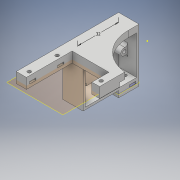
# Autodesk Inventor part: imu_holder
Saved by Autodesk Inventor 2018 (Build 220112000, 112)
## iProperties
Created: 2020-02-18
Part Number: imu_holder
Material: Generic
Document SubType Name: Modeling
Designer: bitbots
Density: 1 g/cm^3
Appearance: Default
Author: bitbots
Autodesk Inventor part; units mm, degrees
ref_plane "YZ Plane" through (0, 0, 0) normal (1, 0, 0) x (0, 1, 0)
ref_plane "XZ Plane" through (0, 0, 0) normal (0, 1, 0) x (-1, 0, 0)
ref_plane "XY Plane" through (0, 0, 0) normal (0, 0, 1) x (1, 0, 0)
sketch "Sketch1" plane through (0, 0, 0) normal (0, 0, 1) x (1, 0, 0)
  arc A0 (-19.5808, 6.2636) -> (-20.1, 4.5766) centre (-17.1, 4.5766) ccw projected
  line L0 (-20.1, -39.6766) -> (-20.1, 4.5766) projected
  arc A1 (-20.1, -39.6766) -> (-19.5808, -41.3636) centre (-17.1, -39.6766) ccw projected
  line L1 (-15.8929, -46.7869) -> (-19.5808, -41.3636) projected
  arc A2 (-15.8929, -46.7869) -> (-13.4121, -48.1) centre (-13.4121, -45.1) ccw projected
  line L2 (13.4121, -48.1) -> (-13.4121, -48.1) projected
  arc A3 (13.4121, -48.1) -> (15.8929, -46.7869) centre (13.4121, -45.1) ccw projected
  line L3 (19.5808, -41.3636) -> (15.8929, -46.7869) projected
  arc A4 (19.5808, -41.3636) -> (20.1, -39.6766) centre (17.1, -39.6766) ccw projected
  line L4 (20.1, 4.5766) -> (20.1, -39.6766) projected
  arc A5 (20.1, 4.5766) -> (19.5808, 6.2636) centre (17.1, 4.5766) ccw projected
  line L5 (15.5953, 12.1246) -> (19.5808, 6.2636) projected
  arc A6 (15.5953, 12.1246) -> (13.9414, 13) centre (13.9414, 11) ccw projected
  line L6 (7.65, 13) -> (13.9414, 13) projected
  arc A7 (9.15, 11.5) -> (7.65, 13) centre (7.65, 11.5) ccw projected
  line L7 (9.15, 11.5) -> (9.15, 10) projected
  arc A8 (9.15, 10) -> (11.5, 7.65) centre (11.5, 10) ccw projected
  line L8 (11.5, 7.65) -> (13.5, 7.65) projected
  arc A9 (14.5, 6.65) -> (13.5, 7.65) centre (13.5, 6.65) ccw projected
  line L9 (14.5, 6.65) -> (14.5, -36.15) projected
  arc A10 (13.5, -37.15) -> (14.5, -36.15) centre (13.5, -36.15) ccw projected
  line L10 (13.5, -37.15) -> (11.5, -37.15) projected
  arc A11 (11.5, -37.15) -> (9.15, -39.5) centre (11.5, -39.5) ccw projected
  line L11 (9.15, -39.5) -> (9.15, -41.5) projected
  arc A12 (8.15, -42.5) -> (9.15, -41.5) centre (8.15, -41.5) ccw projected
  line L12 (8.15, -42.5) -> (-8.15, -42.5) projected
  arc A13 (-9.15, -41.5) -> (-8.15, -42.5) centre (-8.15, -41.5) ccw projected
  line L13 (-9.15, -41.5) -> (-9.15, -39.5) projected
  arc A14 (-9.15, -39.5) -> (-11.5, -37.15) centre (-11.5, -39.5) ccw projected
  line L14 (-11.5, -37.15) -> (-13.5, -37.15) projected
  arc A15 (-14.5, -36.15) -> (-13.5, -37.15) centre (-13.5, -36.15) ccw projected
  line L15 (-14.5, -36.15) -> (-14.5, 6.65) projected
  arc A16 (-13.5, 7.65) -> (-14.5, 6.65) centre (-13.5, 6.65) ccw projected
  line L16 (-13.5, 7.65) -> (-11.5, 7.65) projected
  arc A17 (-11.5, 7.65) -> (-9.15, 10) centre (-11.5, 10) ccw projected
  line L17 (-9.15, 10) -> (-9.15, 11.5) projected
  arc A18 (-7.65, 13) -> (-9.15, 11.5) centre (-7.65, 11.5) ccw projected
  line L18 (-13.9414, 13) -> (-7.65, 13) projected
  arc A19 (-13.9414, 13) -> (-15.5953, 12.1246) centre (-13.9414, 11) ccw projected
  line L19 (-19.5808, 6.2636) -> (-15.5953, 12.1246) projected
  circle A20 centre (17.3, 4) radius 1.35 projected
  circle A21 centre (17.3, -18) radius 1.35 projected
  circle A22 centre (11, -45.3) radius 1.35 projected
  circle A23 centre (-17.3, 4) radius 1.35 projected
  circle A24 centre (-17.3, -18) radius 1.35 projected
  circle A25 centre (-11, -45.3) radius 1.35 projected
  circle A26 centre (17.3, -40) radius 1.35 projected
  circle A27 centre (-17.3, -40) radius 1.35 projected
  line L20 (-17.3, -18) -> (-17.3, -23)
  line L21 (-17.3, -18) -> (-12.3, -18) construction
  line L22 (-17.3, -23) -> (-14.5, -23)
  line L23 (-14.5, -23) -> (-22.5, -23)
  line L24 (-22.5, -23) -> (-22.5, 13.5)
  line L25 (-22.5, 13.5) -> (-14.5, 13.5)
  line L26 (-14.5, 13.5) -> (-14.5, -23)
  line L27 (0, 0) -> (0, -50) construction
  line L28 (14.5, -23) -> (22.5, -23)
  line L29 (22.5, -23) -> (22.5, 13.5)
  line L30 (22.5, 13.5) -> (14.5, 13.5)
  line L31 (14.5, 13.5) -> (14.5, -23)
  line L32 (7.65, 13) -> (-7.65, 13) construction
  line L33 (14.5, 13.5) -> (-14.5, 13.5)
  line L34 (-14.5, 13.5) -> (-14.5, 12.9204)
  line L35 (-14.5, 12.9204) -> (14.5, 12.9204)
  line L36 (14.5, 12.9204) -> (14.5, 13.5)
  dimension "d0" = 5
  dimension "d1" = 90
  dimension "d2" = 8
  dimension "d3" = 36.5
  dimension "d4" = 50
  constraints: 32 end point, 4 parallel, 4 perpendicular, 4 symmetric about line, 3 horizontal, 2 point on line, 2 vertical, 1 point on circle
  measures "d0" distance of L20.start L20.end
  measures "d1" angle of L20 L21
  measures "d2" distance of L24.end L25.end
  measures "d3" distance of L23.end L24.end
  measures "d4" distance of L27.start L27.end
ref_plane "Work Plane1" through (-4.0114, -4.0114, 5) normal (0, 0, 1) x (1, 0, 0)
extrude "Extrusion1" add sketch "Sketch1" along normal up to surface (5 mm away) contours L19 A19 L26 L15 L22 L23 L0 A0 | A0 L0 L23 L24 L25 L26 A19 L19 | L26 L33 L31 A6 L6 A7 L35 A18 L18 A19 | A19 L18 A18 L35 | L30 L29 L28 L4 A5 L5 A6 L31 | A7 L6 A6 L35 | A6 L5 A5 L4 L28 L9 L31
ref_plane "Work Plane2" through (-22.5, 13.5, 2.5) normal (0, 0, 1) x (1, 0, 0)
sketch "Sketch3" plane through (-22.5, 13.5, 2.5) normal (0, 0, 1) x (1, 0, 0)
  line L0 (37, -36.5) -> (37, -0.5796) projected
  line L1 (45, -36.5) -> (37, -36.5) projected
  line L2 (45, 0) -> (45, -36.5) projected
  line L3 (0, 0) -> (45, 0) projected
  line L4 (0, -36.5) -> (0, 0) projected
  line L5 (8, -36.5) -> (0, -36.5) projected
  line L6 (8, -0.5796) -> (8, -36.5) projected
  line L7 (37, -0.5796) -> (8, -0.5796) projected
  circle A0 centre (39.8, -9.5) radius 1.35 projected
  circle A1 centre (39.8, -31.5) radius 1.35 projected
  circle A2 centre (5.2, -9.5) radius 1.35 projected
  circle A3 centre (5.2, -31.5) radius 1.35 projected
  line L8 (2.4, -29.025) -> (8, -29.025)
  line L9 (8, -29.025) -> (8, -33.975)
  line L10 (8, -33.975) -> (2.4, -33.975)
  line L11 (2.4, -33.975) -> (2.4, -29.025)
  line L12 (2.4, -29.025) -> (8, -33.975) construction
  line L13 (8, -29.025) -> (2.4, -33.975) construction
  line L14 (2.4, -7.025) -> (8, -7.025)
  line L15 (8, -7.025) -> (8, -11.975)
  line L16 (8, -11.975) -> (2.4, -11.975)
  line L17 (2.4, -11.975) -> (2.4, -7.025)
  line L18 (2.4, -7.025) -> (8, -11.975) construction
  line L19 (8, -7.025) -> (2.4, -11.975) construction
  line L20 (37, -7.025) -> (42.6, -7.025)
  line L21 (42.6, -7.025) -> (42.6, -11.975)
  line L22 (42.6, -11.975) -> (37, -11.975)
  line L23 (37, -11.975) -> (37, -7.025)
  line L24 (37, -7.025) -> (42.6, -11.975) construction
  line L25 (42.6, -7.025) -> (37, -11.975) construction
  line L26 (37, -29.025) -> (42.6, -29.025)
  line L27 (42.6, -29.025) -> (42.6, -33.975)
  line L28 (42.6, -33.975) -> (37, -33.975)
  line L29 (37, -33.975) -> (37, -29.025)
  line L30 (37, -29.025) -> (42.6, -33.975) construction
  line L31 (42.6, -29.025) -> (37, -33.975) construction
  point P0 (22.5, -13.5)
  dimension "d16" = 5.6
  dimension "d17" = 4.95
  dimension "d18" = 5.6
  dimension "d19" = 4.95
  dimension "d20" = 5.6
  dimension "d21" = 4.95
  dimension "d22" = 5.6
  dimension "d23" = 4.95
  constraints: 48 end point, 8 midpoint, 8 parallel, 4 horizontal, 4 perpendicular
  measures "d16" distance of L9.end L10.end
  measures "d17" distance of L8.end L9.end
  measures "d18" distance of L15.end L16.end
  measures "d19" distance of L14.end L15.end
  measures "d20" distance of L21.end L22.end
  measures "d21" distance of L20.end L21.end
  measures "d22" distance of L27.end L28.end
  measures "d23" distance of L26.end L27.end
extrude "Extrusion2" cut sketch "Sketch3" along normal blind 1.6 contours L0 L26 L27 L28 | L0 L20 L21 L22 | L10 L11 L8 L6 | L6 L16 L17 L14
sketch "Sketch4" plane through (-22.5, 13.5, 0) normal (0, 1, 0) x (1, 0, 0)
  line L0 (0, -5) -> (45, -5) construction
  line L1 (45, 0) -> (45, -5) construction
  line L2 (45, 0) -> (0, 0) construction
  line L3 (0, 0) -> (0, -5) construction
  line L4 (0, 0) -> (0, -5) projected
  line L5 (0, -5) -> (16, -5)
  line L6 (16, -5) -> (16, 29)
  line L7 (16, 29) -> (0, 29)
  line L8 (0, 29) -> (0, -5)
  point P0 (22.5, 0)
  dimension "d26" = 16
  dimension "d27" = 34
  constraints: 8 end point, 2 parallel, 1 horizontal, 1 perpendicular
  measures "d26" distance of L7.end L6.end
  measures "d27" distance of L6.end L5.end
extrude "Extrusion3" add sketch "Sketch4" along normal blind 44
sketch "Sketch5" plane through (-22.5, -23, 0) normal (-1, 0, 0) x (0, 0, 1)
  line L0 (5, 0) -> (5, 80.5) construction
  line L1 (-29, 80.5) -> (5, 80.5) construction
  line L2 (-29, 36.5) -> (-29, 80.5) construction
  line L3 (-29, 36.5) -> (0, 36.5) construction
  line L4 (0, 36.5) -> (0, 0) construction
  line L5 (0, 0) -> (5, 0) construction
  line L6 (-29, 80.5) -> (5, 80.5) construction
  line L7 (5, 80.5) -> (5, 65.6) construction
  line L8 (5, 0) -> (5, 80.5) construction
  line L9 (5, 80.5) -> (19.9, 80.5) construction
  line L10 (5, 65.6) -> (-2.5, 65.6) construction
  line L11 (-2.5, 65.6) -> (-12, 65.6) construction
  line L12 (-12, 65.6) -> (-21.5, 65.6) construction
  line L13 (-0.2, 63.3) -> (-4.8, 63.3)
  line L14 (-4.8, 63.3) -> (-4.8, 67.9)
  line L15 (-4.8, 67.9) -> (-0.2, 67.9)
  line L16 (-0.2, 67.9) -> (-0.2, 63.3)
  line L17 (-0.2, 63.3) -> (-4.8, 67.9) construction
  line L18 (-4.8, 63.3) -> (-0.2, 67.9) construction
  line L19 (-9.7, 63.3) -> (-14.3, 63.3)
  line L20 (-14.3, 63.3) -> (-14.3, 67.9)
  line L21 (-14.3, 67.9) -> (-9.7, 67.9)
  line L22 (-9.7, 67.9) -> (-9.7, 63.3)
  line L23 (-9.7, 63.3) -> (-14.3, 67.9) construction
  line L24 (-14.3, 63.3) -> (-9.7, 67.9) construction
  line L25 (-19.2, 63.3) -> (-23.8, 63.3)
  line L26 (-23.8, 63.3) -> (-23.8, 67.9)
  line L27 (-23.8, 67.9) -> (-19.2, 67.9)
  line L28 (-19.2, 67.9) -> (-19.2, 63.3)
  line L29 (-19.2, 63.3) -> (-23.8, 67.9) construction
  line L30 (-23.8, 63.3) -> (-19.2, 67.9) construction
  point P0 (0, 23)
  dimension "d30" = 14.9
  dimension "d31" = 90
  dimension "d32" = 7.5
  dimension "d33" = 90
  dimension "d34" = 9.5
  dimension "d35" = 9.5
  dimension "d36" = 4.6
  dimension "d37" = 4.6
  dimension "d38" = 4.6
  dimension "d39" = 4.6
  dimension "d40" = 4.6
  dimension "d41" = 4.6
  constraints: 46 end point, 6 midpoint, 6 parallel, 5 perpendicular, 4 horizontal, 2 point on line, 1 collinear
  measures "d30" distance of L0.end L7.end
  measures "d31" angle of L7 L9
  measures "d32" distance of L7.end L10.end
  measures "d33" angle of L7 L10
  measures "d34" distance of L10.end L11.end
  measures "d35" distance of L11.end L12.end
  measures "d36" distance of L14.end L15.end
  measures "d37" distance of L13.end L14.end
  measures "d38" distance of L20.end L21.end
  measures "d39" distance of L19.end L20.end
  measures "d40" distance of L26.end L27.end
  measures "d41" distance of L25.end L26.end
extrude "Extrusion4" cut sketch "Sketch5" against normal blind 9
sketch "Sketch6" plane through (-22.5, 57.5, 0) normal (0, 1, 0) x (1, 0, 0)
  line L0 (0, -5) -> (16, -5) construction
  line L1 (16, -5) -> (16, 29) construction
  line L2 (16, 29) -> (0, 29) construction
  line L3 (0, 29) -> (0, -5) construction
  point P0 (22.5, 0)
sketch "Sketch7" plane through (-6.5, 13.5, 0) normal (1, 0, 0) x (0, 0, -1)
  line L0 (-5, 44) -> (29, 44) projected
  line L1 (-5, 44) -> (-5, 42.2)
  line L2 (-5, 0) -> (-5, 44) projected
  line L3 (-5, 42.2) -> (-3.2, 42.2)
  line L4 (-3.2, 42.2) -> (27.2, 42.2)
  line L5 (27.2, 42.2) -> (27.2, 1.8)
  line L6 (27.2, 1.8) -> (-3.2, 1.8)
  line L7 (-3.2, 1.8) -> (-3.2, 42.2)
  point P0 (0, -13.5)
  dimension "d44" = 1.8
  dimension "d45" = 1.8
  dimension "d46" = 90
  dimension "d47" = 30.4
  dimension "d48" = 40.4
  constraints: 12 end point, 2 parallel, 2 perpendicular, 1 horizontal, 1 point on line
  measures "d44" distance of L0.start L1.end
  measures "d45" distance of L1.end L3.end
  measures "d46" angle of L3 L1
  measures "d47" distance of L5.end L6.end
  measures "d48" distance of L4.end L5.end
extrude "Extrusion5" cut sketch "Sketch7" against normal blind 14
sketch "Sketch8" plane through (-20.5, 13.5, 0) normal (1, 0, 0) x (0, 0, -1)
  line L0 (9.7, 31.4) -> (9.7, 26.8) construction
  line L1 (14.3, 31.4) -> (9.7, 31.4) construction
  line L2 (14.3, 26.8) -> (14.3, 31.4) construction
  line L3 (9.7, 26.8) -> (14.3, 26.8) construction
  line L4 (0.2, 31.4) -> (0.2, 26.8) construction
  line L5 (4.8, 31.4) -> (0.2, 31.4) construction
  line L6 (4.8, 26.8) -> (4.8, 31.4) construction
  line L7 (0.2, 26.8) -> (4.8, 26.8) construction
  line L8 (19.2, 31.4) -> (19.2, 26.8) construction
  line L9 (23.8, 31.4) -> (19.2, 31.4) construction
  line L10 (23.8, 26.8) -> (23.8, 31.4) construction
  line L11 (19.2, 26.8) -> (23.8, 26.8) construction
  line L12 (-3.2, 1.8) -> (-3.2, 42.2) construction
  line L13 (27.2, 1.8) -> (-3.2, 1.8) construction
  line L14 (27.2, 42.2) -> (27.2, 1.8) construction
  line L15 (-3.2, 42.2) -> (27.2, 42.2) construction
  line L16 (27.2, 1.8) -> (-3.2, 1.8) construction
  line L17 (-3.2, 1.8) -> (1.65, 1.8) construction
  line L18 (-3.2, 1.8) -> (1.65, 1.8) construction
  line L19 (1.65, 1.8) -> (1.65, 4.6) construction
  line L20 (1.65, 4.6) -> (21.95, 4.6) construction
  circle A0 centre (1.65, 4.6) radius 1.35
  circle A1 centre (21.95, 4.6) radius 1.35
  circle A2 centre (21.95, 4.6) radius 2.9
  circle A3 centre (1.65, 4.6) radius 2.9
  line L21 (-3.2, 42.2) -> (27.2, 42.2) projected
  line L22 (-3.2, 42.2) -> (11.8, 42.2)
  line L23 (-3.2, 42.2) -> (11.8, 42.2) construction
  line L24 (11.8, 42.2) -> (11.8, 39.5)
  circle A4 centre (11.8, 39.5) radius 1.35
  circle A5 centre (11.8, 39.5) radius 2.6
  point P0 (0, -13.5)
  dimension "d51" = 4.85
  dimension "d52" = 0
  dimension "d53" = 2.8
  dimension "d54" = 90
  dimension "d55" = 20.3
  dimension "d56" = 90
  dimension "d57" = 2.7
  dimension "d58" = 2.7
  dimension "d59" = 5.8
  dimension "d60" = 5.8
  dimension "d61" = 15
  dimension "d62" = 0
  dimension "d63" = 2.7
  dimension "d64" = 2.7
  dimension "d65" = 5.2
  constraints: 14 end point, 6 centre point, 6 coincident, 4 collinear, 3 perpendicular, 2 horizontal
  measures "d51" distance of L12.start L17.end
  measures "d52" distance between parallel lines of L18 L17
  measures "d53" distance of L17.end L19.end
  measures "d54" angle of L19 L17
  measures "d55" distance of L19.end L20.end
  measures "d56" angle of L19 L20
  measures "d57" diameter of A0
  measures "d58" diameter of A1
  measures "d59" diameter of A2
  measures "d60" diameter of A3
  measures "d61" distance of L12.end L22.end
  measures "d62" distance between parallel lines of L23 L22
  measures "d63" distance of L22.end L24.end
  measures "d64" diameter of A4
  measures "d65" diameter of A5
extrude "Extrusion6" cut sketch "Sketch8" against normal up to surface (2 mm away) contours A0 | A1 | A4
sketch "Sketch10" plane through (-20.5, 13.5, 0) normal (1, 0, 0) x (0, 0, -1)
  circle A0 centre (1.65, 4.6) radius 1.35 construction
  circle A1 centre (11.8, 39.5) radius 1.35 projected
  circle A2 centre (21.95, 4.6) radius 1.35 projected
  line L0 (9.7, 31.4) -> (9.7, 26.8) construction
  line L1 (14.3, 31.4) -> (9.7, 31.4) construction
  line L2 (14.3, 26.8) -> (14.3, 31.4) construction
  line L3 (9.7, 26.8) -> (14.3, 26.8) construction
  line L4 (0.2, 31.4) -> (0.2, 26.8) construction
  line L5 (4.8, 31.4) -> (0.2, 31.4) construction
  line L6 (4.8, 26.8) -> (4.8, 31.4) construction
  line L7 (0.2, 26.8) -> (4.8, 26.8) construction
  line L8 (19.2, 31.4) -> (19.2, 26.8) construction
  line L9 (23.8, 31.4) -> (19.2, 31.4) construction
  line L10 (23.8, 26.8) -> (23.8, 31.4) construction
  line L11 (19.2, 26.8) -> (23.8, 26.8) construction
  line L12 (-3.2, 1.8) -> (-3.2, 42.2) construction
  line L13 (27.2, 1.8) -> (-3.2, 1.8) construction
  line L14 (27.2, 42.2) -> (27.2, 1.8) construction
  line L15 (-3.2, 42.2) -> (27.2, 42.2) construction
  circle A3 centre (11.8, 39.5) radius 2.75
  circle A4 centre (21.95, 4.6) radius 2.85
  circle A5 centre (1.65, 4.6) radius 1.35 projected
  circle A6 centre (1.65, 4.6) radius 2.85
  point P0 (0, -13.5)
  dimension "d68" = 5.5
  dimension "d69" = 5.7
  dimension "d70" = 5.7
  constraints: 3 centre point, 3 coincident
  measures "d68" diameter of A3
  measures "d69" diameter of A4
  measures "d70" diameter of A6
extrude "Extrusion7" add sketch "Sketch10" along normal blind 7
sketch "Sketch11" plane through (-22.5, -23, 0) normal (-1, 0, 0) x (0, 0, 1)
  line L0 (5, 0) -> (5, 80.5) construction
  line L1 (-29, 80.5) -> (5, 80.5) construction
  line L2 (-29, 36.5) -> (-29, 80.5) construction
  line L3 (-29, 36.5) -> (0, 36.5) construction
  line L4 (0, 36.5) -> (0, 0) construction
  line L5 (0, 0) -> (5, 0) construction
  line L6 (0.85, 38.6) -> (-4.15, 38.6)
  line L7 (-4.15, 38.6) -> (-4.15, 43.6)
  line L8 (-4.15, 43.6) -> (0.85, 43.6)
  line L9 (0.85, 43.6) -> (0.85, 38.6)
  line L10 (0.85, 38.6) -> (-4.15, 43.6) construction
  line L11 (-4.15, 38.6) -> (0.85, 43.6) construction
  line L12 (-19.45, 38.6) -> (-24.45, 38.6)
  line L13 (-24.45, 38.6) -> (-24.45, 43.6)
  line L14 (-24.45, 43.6) -> (-19.45, 43.6)
  line L15 (-19.45, 43.6) -> (-19.45, 38.6)
  circle A0 centre (-21.95, 41.1) radius 1.35 projected
  line L16 (-19.45, 38.6) -> (-24.45, 43.6) construction
  line L17 (-24.45, 38.6) -> (-19.45, 43.6) construction
  line L18 (-9.3, 73.5) -> (-14.3, 73.5)
  line L19 (-14.3, 73.5) -> (-14.3, 78.5)
  line L20 (-14.3, 78.5) -> (-9.3, 78.5)
  line L21 (-9.3, 78.5) -> (-9.3, 73.5)
  circle A1 centre (-11.8, 76) radius 1.35 projected
  line L22 (-9.3, 73.5) -> (-14.3, 78.5) construction
  line L23 (-14.3, 73.5) -> (-9.3, 78.5) construction
  circle A2 centre (-1.65, 41.1) radius 1.35 construction
  point P0 (0, 23)
  dimension "d73" = 5
  dimension "d74" = 5
  dimension "d75" = 5
  dimension "d76" = 5
  dimension "d77" = 5
  dimension "d78" = 5
  constraints: 36 end point, 6 parallel, 5 midpoint, 3 horizontal, 3 perpendicular, 1 coincident
  measures "d73" distance of L7.end L8.end
  measures "d74" distance of L6.end L7.end
  measures "d75" distance of L13.end L14.end
  measures "d76" distance of L12.end L13.end
  measures "d77" distance of L19.end L20.end
  measures "d78" distance of L18.end L19.end
extrude "Extrusion8" cut sketch "Sketch11" against normal blind 1.6
sketch "Sketch12" plane through (-22.5, -23, 0) normal (-1, 0, 0) x (0, 0, 1)
  line L0 (-14.3, 78.5) -> (-9.3, 78.5) construction
  line L1 (5, 0) -> (5, 80.5) construction
  line L2 (-29, 80.5) -> (5, 80.5) construction
  line L3 (-29, 36.5) -> (-29, 80.5) construction
  line L4 (-29, 36.5) -> (0, 36.5) construction
  line L5 (0, 36.5) -> (0, 0) construction
  line L6 (0, 0) -> (5, 0) construction
  line L7 (5, 36.5) -> (5, 80.5) construction
  line L8 (5, 80.5) -> (5, 48.5) construction
  line L9 (-9.3, 78.5) -> (-9.3, 73.5) projected
  line L10 (-9.3, 73.5) -> (-14.3, 73.5) projected
  line L11 (-14.3, 73.5) -> (-14.3, 78.5) projected
  point P0 (0, 23)
  dimension "d81" = 32
  constraints: 2 end point, 1 point on line
  measures "d81" distance of L1.end L8.end
ref_plane "Work Plane3" through (-24.5, -41.5055, -34.0037) normal (1, 0, 0) x (0, 1, 0)
sketch "Sketch14" plane through (-6.5, 13.5, -29) normal (0, 0, -1) x (-1, 0, 0)
  line L0 (23, -53) -> (5.6855, -75.3568) construction
  line L1 (23, -53) -> (23, 42.8925) construction
  arc A0 (23, 42.8925) -> (22.4142, 44.3067) centre (21, 42.8925) ccw construction
  line L2 (22.4142, 44.3067) -> (9.3067, 57.4142) construction
  arc A1 (9.3067, 57.4142) -> (7.8925, 58) centre (7.8925, 56) ccw construction
  line L3 (7.8925, 58) -> (-5.1716, 58) construction
  arc A2 (-5.1716, 58) -> (-6.5858, 57.4142) centre (-5.1716, 56) ccw construction
  line L4 (-6.5858, 57.4142) -> (-11.4142, 52.5858) construction
  arc A3 (-12.8284, 52) -> (-11.4142, 52.5858) centre (-12.8284, 54) ccw construction
  line L5 (-12.8284, 52) -> (-127, 52) construction
  line L6 (-127, 52) -> (-127, -73) construction
  line L7 (-127, -73) -> (-121.462, -73) construction
  arc A4 (-120.54, -73.0426) -> (-121.462, -73) centre (-121.462, -83) ccw construction
  line L8 (-120.54, -73.0426) -> (-67.46, -77.9574) construction
  arc A5 (-67.46, -77.9574) -> (-66.538, -78) centre (-66.538, -68) ccw construction
  line L9 (-66.538, -78) -> (-1.0877, -78) construction
  arc A6 (-1.0877, -78) -> (5.6855, -75.3568) centre (-1.0877, -68) ccw construction
  circle A7 centre (-73, 42) radius 2.5 construction
  circle A8 centre (-73, -13) radius 2.5 construction
  circle A9 centre (6, 39) radius 2.5 construction
  circle A10 centre (-11, 47) radius 2.5 construction
  circle A11 centre (-35.5, 47) radius 2.5 construction
  circle A12 centre (-60, 47) radius 2.5 construction
  circle A13 centre (-111, -69) radius 2.5 construction
  circle A14 centre (-77.1448, -72.1347) radius 2.5 construction
  circle A15 centre (-60, -73) radius 2.5 construction
  circle A16 centre (-35.5, -73) radius 2.5 construction
  circle A17 centre (-11, -73) radius 2.5 construction
  circle A18 centre (10.8, -53.5) radius 1.025 construction
  circle A19 centre (10.8, -31.5) radius 1.025 construction
  circle A20 centre (10.8, -9.5) radius 1.025 construction
  circle A21 centre (-23.8, -9.5) radius 1.025 construction
  circle A22 centre (-23.8, -31.5) radius 1.025 construction
  circle A23 centre (-23.8, -53.5) radius 1.025 construction
  circle A24 centre (4.5, -58.8) radius 1.025 construction
  circle A25 centre (-17.5, -58.8) radius 1.025 construction
  circle A26 centre (-73, -68) radius 2.5 construction
  line L10 (-28, 43) -> (-65.5, 43) construction
  arc A27 (-26, 41) -> (-28, 43) centre (-28, 41) ccw construction
  line L11 (-26, 41) -> (-26, 22) construction
  arc A28 (-28, 20) -> (-26, 22) centre (-28, 22) ccw construction
  line L12 (-28, 20) -> (-65.5, 20) construction
  arc A29 (-67.5, 22) -> (-65.5, 20) centre (-65.5, 22) ccw construction
  line L13 (-67.5, 22) -> (-67.5, 41) construction
  arc A30 (-65.5, 43) -> (-67.5, 41) centre (-65.5, 41) ccw construction
  line L14 (-118, 46.5) -> (-80.5, 46.5) construction
  arc A31 (-78.5, 44.5) -> (-80.5, 46.5) centre (-80.5, 44.5) ccw construction
  line L15 (-78.5, 44.5) -> (-78.5, 22) construction
  arc A32 (-80.5, 20) -> (-78.5, 22) centre (-80.5, 22) ccw construction
  line L16 (-80.5, 20) -> (-118, 20) construction
  arc A33 (-120, 22) -> (-118, 20) centre (-118, 22) ccw construction
  line L17 (-120, 22) -> (-120, 44.5) construction
  arc A34 (-118, 46.5) -> (-120, 44.5) centre (-118, 44.5) ccw construction
  line L18 (-111.9569, 15) -> (-80.5, 15) construction
  arc A35 (-78.5, 13) -> (-80.5, 15) centre (-80.5, 13) ccw construction
  line L19 (-78.5, 13) -> (-78.5, -21.3542) construction
  arc A36 (-81.975, -22.7049) -> (-78.5, -21.3542) centre (-80.5, -21.3542) ccw construction
  line L20 (-81.975, -22.7049) -> (-113.4319, 11.6494) construction
  arc A37 (-111.9569, 15) -> (-113.4319, 11.6494) centre (-111.9569, 13) ccw construction
  line L21 (-86.5431, -30) -> (-118, -30) construction
  arc A38 (-120, -28) -> (-118, -30) centre (-118, -28) ccw construction
  line L22 (-120, -28) -> (-120, 6.3542) construction
  arc A39 (-116.525, 7.7049) -> (-120, 6.3542) centre (-118, 6.3542) ccw construction
  line L23 (-116.525, 7.7049) -> (-85.0681, -26.6494) construction
  arc A40 (-86.5431, -30) -> (-85.0681, -26.6494) centre (-86.5431, -28) ccw construction
  line L24 (-64.025, 7.7049) -> (-32.5681, -26.6494) construction
  arc A41 (-34.0431, -30) -> (-32.5681, -26.6494) centre (-34.0431, -28) ccw construction
  line L25 (-34.0431, -30) -> (-65.5, -30) construction
  arc A42 (-67.5, -28) -> (-65.5, -30) centre (-65.5, -28) ccw construction
  line L26 (-67.5, -28) -> (-67.5, 6.3542) construction
  arc A43 (-64.025, 7.7049) -> (-67.5, 6.3542) centre (-65.5, 6.3542) ccw construction
  line L27 (-29.475, -22.7049) -> (-60.9319, 11.6494) construction
  arc A44 (-59.4569, 15) -> (-60.9319, 11.6494) centre (-59.4569, 13) ccw construction
  line L28 (-59.4569, 15) -> (-28, 15) construction
  arc A45 (-26, 13) -> (-28, 15) centre (-28, 13) ccw construction
  line L29 (-26, 13) -> (-26, -21.3542) construction
  arc A46 (-29.475, -22.7049) -> (-26, -21.3542) centre (-28, -21.3542) ccw construction
  line L30 (-67.5, -67) -> (-67.5, -37) construction
  arc A47 (-65.5, -35) -> (-67.5, -37) centre (-65.5, -37) ccw construction
  line L31 (-65.5, -35) -> (-28, -35) construction
  arc A48 (-26, -37) -> (-28, -35) centre (-28, -37) ccw construction
  line L32 (-26, -37) -> (-26, -67) construction
  arc A49 (-28, -69) -> (-26, -67) centre (-28, -67) ccw construction
  line L33 (-65.5, -69) -> (-28, -69) construction
  arc A50 (-67.5, -67) -> (-65.5, -69) centre (-65.5, -67) ccw construction
  line L34 (5.0579, 54.1421) -> (18.4929, 40.7071) construction
  arc A51 (18.4929, 39.2929) -> (18.4929, 40.7071) centre (17.7858, 40) ccw construction
  line L35 (18.4929, 39.2929) -> (17.7363, 38.5363) construction
  arc A52 (16.3221, 38.5363) -> (17.7363, 38.5363) centre (17.0292, 39.2434) ccw construction
  line L36 (16.3221, 38.5363) -> (2.887, 51.9713) construction
  arc A53 (2.887, 53.3855) -> (2.887, 51.9713) centre (3.5942, 52.6784) ccw construction
  line L37 (2.887, 53.3855) -> (3.6437, 54.1421) construction
  arc A54 (5.0579, 54.1421) -> (3.6437, 54.1421) centre (4.3508, 53.435) ccw construction
  line L38 (-120, -63) -> (-120, -37) construction
  arc A55 (-118, -35) -> (-120, -37) centre (-118, -37) ccw construction
  line L39 (-118, -35) -> (-80.5, -35) construction
  arc A56 (-78.5, -37) -> (-80.5, -35) centre (-80.5, -37) ccw construction
  line L40 (-78.5, -37) -> (-78.5, -68.3661) construction
  arc A57 (-78.636, -68.4231) -> (-78.5, -68.3661) centre (-80.5, -63.7835) ccw construction
  arc A58 (-78.636, -68.4231) -> (-80.5765, -70.0796) centre (-77.1448, -72.1347) ccw construction
  arc A59 (-82.4767, -71.0434) -> (-80.5765, -70.0796) centre (-82.2923, -69.052) ccw construction
  line L41 (-82.4767, -71.0434) -> (-105.5584, -68.9063) construction
  arc A60 (-107.2493, -67.6098) -> (-105.5584, -68.9063) centre (-105.374, -66.9148) ccw construction
  arc A61 (-107.2493, -67.6098) -> (-111, -65) centre (-111, -69) ccw construction
  line L42 (-111, -65) -> (-118, -65) construction
  arc A62 (-120, -63) -> (-118, -65) centre (-118, -63) ccw construction
  line L43 (0, 43) -> (-19, 43) construction
  arc A63 (2, 41) -> (0, 43) centre (0, 41) ccw construction
  line L44 (2, 41) -> (2, 39) construction
  arc A64 (2, 39) -> (6, 35) centre (6, 39) ccw construction
  line L45 (6, 35) -> (11, 35) construction
  arc A65 (16, 30) -> (11, 35) centre (11, 30) ccw construction
  line L46 (16, 30) -> (16, -3.5) construction
  arc A66 (14, -5.5) -> (16, -3.5) centre (14, -3.5) ccw construction
  line L47 (14, -5.5) -> (10, -5.5) construction
  arc A67 (10, -5.5) -> (10, -7.5) centre (10, -7.5) ccw construction
  line L48 (8, -7.5) -> (8, -11.5) construction
  arc A68 (8, -11.5) -> (10, -13.5) centre (10, -11.5) ccw construction
  line L49 (10, -13.5) -> (14, -13.5) construction
  arc A69 (16, -15.5) -> (14, -13.5) centre (14, -15.5) ccw construction
  line L50 (16, -15.5) -> (16, -25.5) construction
  arc A70 (14, -27.5) -> (16, -25.5) centre (14, -25.5) ccw construction
  line L51 (14, -27.5) -> (10, -27.5) construction
  arc A71 (10, -27.5) -> (10, -29.5) centre (10, -29.5) ccw construction
  line L52 (8, -29.5) -> (8, -33.5) construction
  arc A72 (8, -33.5) -> (10, -35.5) centre (10, -33.5) ccw construction
  line L53 (10, -35.5) -> (14, -35.5) construction
  arc A73 (16, -37.5) -> (14, -35.5) centre (14, -37.5) ccw construction
  line L54 (16, -37.5) -> (16, -47.5) construction
  arc A74 (14, -49.5) -> (16, -47.5) centre (14, -47.5) ccw construction
  line L55 (14, -49.5) -> (10, -49.5) construction
  arc A75 (10, -49.5) -> (10, -51.5) centre (10, -51.5) ccw construction
  line L56 (8, -51.5) -> (8, -54.5) construction
  arc A76 (6.5, -56) -> (8, -54.5) centre (6.5, -54.5) ccw construction
  line L57 (6.5, -56) -> (-19.5, -56) construction
  arc A77 (-21, -54.5) -> (-19.5, -56) centre (-19.5, -54.5) ccw construction
  line L58 (-21, -54.5) -> (-21, 41) construction
  arc A78 (-19, 43) -> (-21, 41) centre (-19, 41) ccw construction
  line L59 (0, 0) -> (0, 44) projected
  line L60 (0, 44) -> (8, 44)
  line L61 (0, 44) -> (16, 44) projected
  line L62 (0, 44) -> (8, 44) construction
  line L63 (8, 44) -> (16, 36)
  line L64 (16, 0) -> (16, 44) projected
  line L65 (16, 36) -> (16, 28)
  line L66 (16, 28) -> (0, 28)
  line L67 (0, 28) -> (0, 44)
  point P0 (-6.5, -13.5)
  dimension "d88" = 8
  dimension "d89" = 0
  dimension "d90" = 135
  dimension "d91" = 8
  dimension "d92" = 135
  dimension "d94" = 90
  constraints: 12 end point, 4 collinear, 1 horizontal, 1 perpendicular, 1 point on line, 3 other
  measures "d88" distance of L59.end L60.end
  measures "d89" distance between parallel lines of L60 L62
  measures "d90" angle of L60 L63
  measures "d91" distance of L63.end L65.end
  measures "d92" angle of L63 L65
  measures "d94" angle of L65 L66
ref_plane "Work Plane4" through (-29.6931, -64.713, -34) normal (0, 0, 1) x (1, 0, 0)
extrude "Extrusion10" add sketch "Sketch14" along normal up to surface (5 mm away) contours L59 L60 L63 L64 L66
sketch "Sketch15" plane through (22.5, -23, 0) normal (1, 0, 0) x (0, 0, -1)
  line L0 (-5, 36.5) -> (-5, 0) projected
  line L1 (0, 0) -> (-5, 0) projected
  line L2 (0, 0) -> (0, 36.5) projected
  line L3 (0, 36.5) -> (-5, 36.5) projected
  point P0 (0, 23)
extrude "Extrusion11" cut sketch "Sketch15" against normal blind 2
sketch "Sketch18" plane through (-6.5, 41.5, -34) normal (0, 0, -1) x (-1, 0, 0)
  circle A0 centre (6, 11) radius 1.4 construction
  circle A1 centre (6, 11) radius 1.35
  circle A2 centre (6, 11) radius 1.4 construction
  point P0 (-6.5, -41.5)
  dimension "d106" = 2.7
  constraints: 2 centre point, 2 coincident
  measures "d106" diameter of A1
extrude "Extrusion14" cut sketch "Sketch18" against normal up to surface (6.8 mm away)
ref_plane "Work Plane5" through (-6.5, 41.5, -31) normal (0, 0, -1) x (-1, 0, 0)
sketch "Sketch19" plane through (-6.5, 41.5, -31) normal (0, 0, -1) x (-1, 0, 0)
  circle A0 centre (6, 11) radius 1.35 construction
  circle A1 centre (6, 11) radius 1.35 construction
  line L0 (8.5, 8.5) -> (3.5, 8.5)
  line L1 (3.5, 8.5) -> (3.5, 13.5)
  line L2 (3.5, 13.5) -> (8.5, 13.5)
  line L3 (8.5, 13.5) -> (8.5, 8.5)
  circle A2 centre (6, 11) radius 1.35 projected
  line L4 (8.5, 8.5) -> (3.5, 13.5) construction
  line L5 (3.5, 8.5) -> (8.5, 13.5) construction
  line L6 (0, 14.2) -> (0, -26.2) construction
  line L7 (0, 8.5) -> (3.5, 8.5)
  line L8 (3.5, 8.5) -> (3.5, 13.5)
  line L9 (3.5, 13.5) -> (0, 13.5)
  line L10 (0, 13.5) -> (0, 8.5)
  point P0 (-6.5, -41.5)
  dimension "d110" = 5
  dimension "d111" = 5
  constraints: 20 end point, 4 parallel, 2 horizontal, 2 midpoint, 2 perpendicular, 1 point on line
  measures "d110" distance of L1.end L2.end
  measures "d111" distance of L0.end L1.end
extrude "Extrusion15" cut sketch "Sketch19" against normal blind 1.6
fillet "Fillet1" radius 2 6 edges at (-17, 55.7, -11.278) (-17, 55.7, -12.322) (-17, 15.3, -2.1815) (-17, 15.3, -1.1185) (-17, 15.3, -21.4185) (-17, 15.3, -22.4815)
sketch "Sketch20" plane through (-22.5, -23, 0) normal (-1, 0, 0) x (0, 0, 1)
  circle A0 centre (-1.65, 41.1) radius 1.35 projected
  line L0 (0.85, 38.6) -> (-4.15, 38.6) projected
  line L1 (0.85, 43.6) -> (0.85, 38.6) projected
  line L2 (-4.15, 43.6) -> (0.85, 43.6) projected
  line L3 (-4.15, 38.6) -> (-4.15, 43.6) projected
  circle A1 centre (-21.95, 41.1) radius 1.35 projected
  line L4 (-19.45, 38.6) -> (-24.45, 38.6) projected
  line L5 (-19.45, 43.6) -> (-19.45, 38.6) projected
  line L6 (-24.45, 43.6) -> (-19.45, 43.6) projected
  line L7 (-24.45, 38.6) -> (-24.45, 43.6) projected
  line L8 (-24.45, 43.6) -> (-29, 43.6)
  line L9 (-29, 36.5) -> (-29, 64.5) projected
  line L10 (-27.2, 78.7) -> (-27.2, 38.3) projected
  line L11 (-27.2, 43.6) -> (2.8, 43.6)
  line L12 (2.8, 43.6) -> (2.8, 54.6)
  line L13 (2.8, 54.6) -> (-27.2, 54.6)
  line L14 (-27.2, 54.6) -> (-27.2, 43.6)
  point P0 (0, 23)
  dimension "d115" = 30
  dimension "d116" = 11
  constraints: 10 end point, 3 point on line, 2 horizontal, 2 parallel, 1 perpendicular
  measures "d115" distance of L13.end L12.end
  measures "d116" distance of L12.end L11.end
extrude "Extrusion16" cut sketch "Sketch20" against normal blind 0.5 contours L2 L11 L6 L8 L10 L13 L12
sketch "Sketch21" plane through (-22, -23, 0) normal (-1, 0, 0) x (0, 0, 1)
  line L0 (2.8, 43.6) -> (0.85, 43.6) construction
  line L1 (2.8, 54.6) -> (2.8, 43.6) construction
  line L2 (-27.2, 54.6) -> (2.8, 54.6) construction
  line L3 (-27.2, 43.6) -> (-27.2, 54.6) construction
  line L4 (-24.45, 43.6) -> (-27.2, 43.6) construction
  line L5 (-19.45, 43.6) -> (-24.45, 43.6) construction
  line L6 (-4.15, 43.6) -> (-19.45, 43.6) construction
  line L7 (0.85, 43.6) -> (-4.15, 43.6) construction
  line L8 (-24.45, 43.6) -> (-27.2, 43.6) construction
  line L9 (-27.2, 43.6) -> (-27.2, 45.1) construction
  line L10 (-27.2, 43.6) -> (-27.2, 54.6) construction
  line L11 (-27.2, 45.1) -> (-25.2, 45.1)
  line L12 (-25.2, 45.1) -> (-25.2, 53.1)
  line L13 (-25.2, 53.1) -> (-27.2, 53.1)
  line L14 (-27.2, 53.1) -> (-27.2, 45.1)
  point P0 (0, 23)
  dimension "d119" = 1.5
  dimension "d120" = 2
  dimension "d121" = 8
  constraints: 10 end point, 2 parallel, 1 horizontal, 1 perpendicular, 1 point on line
  measures "d119" distance of L3.start L9.end
  measures "d120" distance of L13.end L12.end
  measures "d121" distance of L12.end L11.end
extrude "Extrusion17" cut sketch "Sketch21" against normal up to surface (1.5 mm away)
sketch "Sketch23" plane through (-13.5, 13.5, 0) normal (1, 0, 0) x (0, 0, -1)
  arc A0 (4.461, 4.1299) -> (-1.161, 4.1299) centre (1.65, 4.6) ccw projected
  circle A1 centre (1.65, 4.6) radius 1.35 projected
  arc A2 (24.761, 4.1299) -> (19.139, 4.1299) centre (21.95, 4.6) ccw projected
  circle A3 centre (21.95, 4.6) radius 1.35 projected
  line L0 (26.7336, 1.8) -> (17.1664, 1.8) projected
  arc A4 (24.761, 4.1299) -> (26.7336, 1.8) centre (26.7336, 3.8) ccw projected
  arc A5 (17.1664, 1.8) -> (19.139, 4.1299) centre (17.1664, 3.8) ccw projected
  line L1 (6.4336, 1.8) -> (-3.1336, 1.8) projected
  arc A6 (4.461, 4.1299) -> (6.4336, 1.8) centre (6.4336, 3.8) ccw projected
  arc A7 (-3.1336, 1.8) -> (-1.161, 4.1299) centre (-3.1336, 3.8) ccw projected
  point P0 (0, -13.5)
extrude "Extrusion19" cut sketch "Sketch23" against normal blind 1.5
sketch "Sketch24" plane through (-6.5, 13.5, 5) normal (0, 1, 0) x (1, 0, 0)
  line L0 (27, 0) -> (27, 5) projected
  line L1 (27, 5) -> (0, 5) projected
  line L2 (0, 5) -> (0, 0) projected
  line L3 (0, 0) -> (27, 0) projected
  point P0 (6.5, 5)
extrude "Extrusion20" add sketch "Sketch24" along normal up to surface (1.8 mm away)
fillet "Fillet2" [suppressed]
sketch "Sketch25" plane through (14.5, -23, 0) normal (0, -1, 0) x (1, 0, 0)
  line L0 (6, 0) -> (6, 5) projected
  line L1 (6, 5) -> (0, 5) projected
  line L2 (0, 0) -> (0, 5) projected
  line L3 (0, 0) -> (6, 0) projected
  point P0 (-14.5, 0)
extrude "Extrusion21" cut sketch "Sketch25" against normal blind 22.5
chamfer "Chamfer1" [suppressed]
sketch "Sketch27" plane through (-6.5, 15.3, 0) normal (0, 1, 0) x (1, 0, 0)
  line L0 (0, -5) -> (0, -3.2) projected
  line L1 (0, -5) -> (0, -3.2)
  line L2 (0, -3.2) -> (27, -3.2)
  line L3 (27, -5) -> (27, 0) projected
  line L4 (27, -5) -> (27, -3.2)
  line L5 (22.45, -2.5) -> (25.15, -2.5) projected
  line L6 (0, -5) -> (27, -5) projected
  line L7 (27, -5) -> (0, -5)
  point P0 (6.5, 0)
  constraints: 8 end point, 2 collinear, 2 perpendicular, 1 point on line
extrude "Extrusion23" add sketch "Sketch27" along normal blind 4
fillet "Fillet3" radius 30 1 edges at (-6.5, 19.3, 4.1)
sketch "Sketch29" plane through (-14.5, 12.9204, 5) normal (0, 0, 1) x (1, 0, 0)
  line L0 (29, -13.4204) -> (35, -13.4204) projected
  line L1 (35, -13.4204) -> (35, 6.3796) projected
  arc A0 (8, 36.2292) -> (35, 6.3796) centre (38, 36.2292) ccw projected
  line L2 (8, 36.2292) -> (8, 44.5796) projected
  line L3 (-8, 44.5796) -> (8, 44.5796) projected
  line L4 (-8, -35.9204) -> (-8, 44.5796) projected
  line L5 (0, -35.9204) -> (-8, -35.9204) projected
  line L6 (0, 0) -> (0, -35.9204) projected
  line L7 (29, 0) -> (0, 0) projected
  line L8 (29, -13.4204) -> (29, 0) projected
  circle A1 centre (31.8, -8.9204) radius 1.35 projected
  circle A2 centre (-2.8, -8.9204) radius 1.35 projected
  circle A3 centre (-2.8, -30.9204) radius 1.35 projected
  point P0 (14.5, -12.9204)
extrude "Extrusion24" add sketch "Sketch29" along normal blind 3.2
equation "\"d36\" = button_width"
equation "\"d37\" = button_width"
equation "\"d38\" = button_width"
equation "\"d39\" = button_width"
equation "\"d40\" = button_width"
equation "\"d41\" = button_width"
equation "\"button_width\" = 4.6"
body "Solid1"
